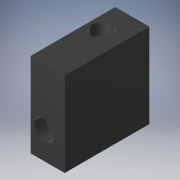
# Autodesk Inventor part: BT406_trajan20_21
Saved by Autodesk Inventor 2022.2 (Build 262287000, 287)
## iProperties
Company: HTBLA Kaindorf
RuleStatus: InUse
Created: 2022-08-23
Part Number: BT406_trajan20_21
Project: Zeichenmaschine_v2
Material: Kunststoff, undurchsichtig Schwarz
Description: Ecken
Document SubType Name: Modeling
Designer: trajan20
Density: 0.952 g/cm^3
Appearance: Glatt - Schwarz
Mass: 2.66244 g
Surface Area: 23.573 cm^2
Volume: 2.79668 cm^3
AfterDocNew0: iProperties-Editor_aufrufen
Author: jan
Keywords: 2021
Autodesk Inventor part; units mm, degrees
ref_plane "YZ Plane" through (0, 0, 0) normal (1, 0, 0) x (0, 1, 0)
ref_plane "XZ Plane" through (0, 0, 0) normal (0, 1, 0) x (-1, 0, 0)
ref_plane "XY Plane" through (0, 0, 0) normal (0, 0, 1) x (1, 0, 0)
sketch "Skizze3" plane through (0, 0, 0) normal (0, 1, 0) x (-1, 0, 0)
  line L0 (5, -5) -> (5, -25)
  line L1 (5, -25) -> (0, -25)
  line L2 (0, -25) -> (0, 0)
  line L3 (0, 0) -> (5, -5)
  dimension "d7" = 5
  dimension "d11" = 25
  dimension "d12" = 20
  constraints: 8 end point, 2 perpendicular, 1 vertical
  measures "d7" distance between parallel lines of L2 L0
  measures "d11" distance from line of L1 L2.end
  measures "d12" distance of L0.start L0.end
extrude "Extrusion3" add sketch "Skizze3" along normal blind 8
sketch "Skizze4" plane through (0, 0, 0) normal (1, 0, 0) x (0, 0, -1)
  line L0 (-0.7299, 4) -> (5.994, 4) construction
  line L1 (0, 0) -> (0, 8) projected
  point P0 (17, 4)
  point P1 (0, 4)
  dimension "d10" = 17
  constraints: 2 end point, 2 point on line, 1 horizontal, 1 midpoint
  measures "d10" distance from line of L1 point (17, 4)
hole "Bohrung1" at (0, 4, -17) direction (-1, 0, 0) diameter 3.4 end through all counterbore diameter 6 counterbore depth 3.4
chamfer "Fase1" distance 2 angle 45 1 edges at (-5, 4, -25)
mirror "Spiegeln1" about plane through (-5, 0, -5) normal (-0.7071068, 0, 0.7071068) of "Extrusion3", "Bohrung1", "Fase1"
sketch "Skizze5" plane through (0, 0, -25) normal (1, 0, 0) x (0, 0, -1)
  line L0 (-25, 8) -> (0, 8) projected
  line L1 (-25, 0) -> (-25, 8) projected
  line L2 (-25, 8) -> (0, 8)
  line L3 (0, 8) -> (0, 10)
  line L4 (0, 10) -> (-25, 10)
  line L5 (-25, 10) -> (-25, 8)
  dimension "d23" = 2
  constraints: 8 end point, 2 parallel, 1 horizontal, 1 perpendicular
  measures "d23" distance between parallel lines of L4 L0
extrude "Extrusion4" add sketch "Skizze5" against normal blind 25
equation "\"d12\" = d11 - d7"
